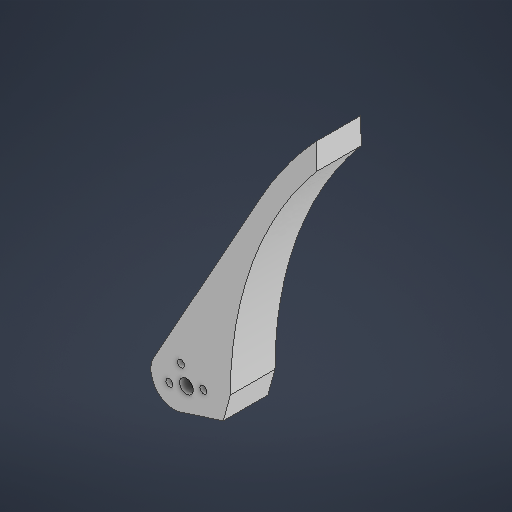
# Autodesk Inventor part: направление
Saved by Autodesk Inventor 2025 (Build 290162000, 162)
## iProperties
Created: 2025-11-04
Part Number: направление
Material: Типовые
Document SubType Name: Modeling
Designer: GameHD
Density: 1 g/cm^3
Appearance: По умолчанию
Author: GameHD
Autodesk Inventor part; units mm, degrees
ref_plane "YZ Plane" through (0, 0, 0) normal (1, 0, 0) x (0, 1, 0)
ref_plane "XZ Plane" through (0, 0, 0) normal (0, 1, 0) x (-1, 0, 0)
ref_plane "XY Plane" through (0, 0, 0) normal (0, 0, 1) x (1, 0, 0)
sketch "Эскиз1" plane through (0, 0, 0) normal (0, 0, 1) x (1, 0, 0)
  circle A0 centre (0, 0) radius 165
  circle A1 centre (0, 0) radius 172.834
  line L0 (-125, 0) -> (-126.5392, 117.7261)
  line L1 (-132.7592, 119.5177) -> (-197.8467, 76.6552)
  line L2 (-165, 0) -> (-153, 0) construction
  line L3 (-134.7038, 9.8338) -> (-172.765, -2.5204) projected
  line L4 (-165, 0) -> (-172.8154, -2.5368)
  point P0 (-172.834, 0)
  point P1 (-126.3868, 106.0725)
  point P2 (-123, 114.4334)
  point P3 (-172.8149, -2.5694)
  dimension "d0" = 330
  dimension "d1" = 345.668
  dimension "d2" = 40
  constraints: 8 end point, 4 point on circle, 2 coincident, 1 centre point, 1 collinear, 1 horizontal, 1 tangent, 3 other
  measures "d1" diameter of A1
  measures "d2" distance of L2.start L0.start
extrude "Выдавливание1" add sketch "Эскиз1" along normal blind 20 contours L3 L4 A1 L0 A0 picked at (-133.2989, 101.385)
sketch "Эскиз2" plane through (0, 0, 0) normal (0, 0, -1) x (-1, 0, 0)
  arc A0 (172.8154, -2.5368) -> (126.5392, 117.7261) centre (0, 0) ccw projected
  arc A1 (165, 0) -> (126.3868, 106.0725) centre (0, 0) ccw projected
  circle A2 centre (0, 0) radius 168.917
  line L0 (172.8154, -2.5368) -> (165, 0) projected
  circle A3 centre (184.6734, -6.3858) radius 2.1
  line L1 (178.0154, -4.2246) -> (172.8154, -2.5368)
  line L2 (160.1198, 6.946) -> (198.8648, -5.6302)
  line L3 (182.8662, -5.7992) -> (187.0032, 6.946)
  line L4 (178.0154, -4.2246) -> (198.192, -10.7737)
  line L5 (184.6734, -6.3858) -> (189.5243, -7.9603)
  line L6 (189.5243, -7.9603) -> (192.7095, 1.8528)
  point P0 (184.4408, -0.9483)
  point P1 (172.8109, 2.8266)
  point P2 (176.018, -3.5763)
  point P3 (182.676, -5.7374)
  point P4 (183.1424, -4.9484)
  point P5 (164.9119, 5.3905)
  point P6 (186.6708, -7.0341)
  point P7 (191.0988, -3.1094)
  dimension "d8" = 337.834
  dimension "d11" = 4.2
  dimension "d18" = 5.1
  constraints: 12 end point, 2 centre point, 2 perpendicular, 1 coincident, 1 collinear, 1 parallel, 1 point on line
  measures "d8" diameter of A2
  measures "d11" diameter of A3
  measures "d18" distance of L5.start L5.end
extrude "Выдавливание2" add sketch "Эскиз2" against normal up to surface (20 mm away) contours L0 A2 L2 A0 | A0 L2 L3 A3 L4 L1 | L0 A1 L2 A2 | L2 L6 L4 A3 L3 picked at (166.282, 2.7097)
sketch "Эскиз3" plane through (0, 0, 20) normal (0, 0, 1) x (1, 0, 0)
  arc A0 (-126.3868, 106.0725) -> (-165, 0) centre (0, 0) ccw projected
  line L0 (-126.3868, 106.0725) -> (-126.5392, 117.7261) projected
  arc A1 (-126.5392, 117.7261) -> (-172.8109, 2.8266) centre (0, 0) ccw projected
  line L1 (-191.0988, -3.1094) -> (-172.8109, 2.8266) projected
  line L2 (-189.5243, -7.9603) -> (-191.0988, -3.1094) projected
  line L3 (-186.6708, -7.0341) -> (-189.5243, -7.9603) projected
  arc A2 (-182.676, -5.7374) -> (-186.6708, -7.0341) centre (-184.6734, -6.3858) ccw projected
  line L4 (-165, 0) -> (-182.676, -5.7374) projected
  circle A3 centre (-184.6734, -6.3858) radius 3.1
  arc A4 (-126.5392, 117.7261) -> (-172.8109, 2.8266) centre (0, 0) ccw projected
  line L5 (-184.6734, -6.3858) -> (-194.1849, -9.4731)
  line L6 (-194.1849, -9.4731) -> (-195.7594, -4.6222)
  line L7 (-195.7594, -4.6222) -> (-191.0988, -3.1094)
  circle A5 centre (-184.6734, -6.3858) radius 11
  circle A6 centre (-184.6734, -6.3858) radius 9.5
  circle A7 centre (-184.6734, -6.3858) radius 6.5
  line L8 (-190.8559, -8.3925) -> (-193.7093, -9.3187)
  circle A8 centre (-192.2826, -8.8556) radius 1.6
  circle A9 centre (-182.2036, -13.995) radius 1.6
  circle A10 centre (-177.0642, -3.9159) radius 1.6
  circle A11 centre (-187.1433, 1.2234) radius 1.6
  line L9 (-192.2826, -8.8556) -> (-199.8918, -11.3255)
  line L10 (-199.8918, -11.3255) -> (-201.4663, -6.4746)
  line L11 (-201.4663, -6.4746) -> (-191.0988, -3.1094)
  line L12 (-201.4663, -6.4746) -> (-195.8644, -23.7333)
  line L13 (-172.8109, 2.8266) -> (-166.0857, -17.8924)
  line L14 (-184.6734, -6.3858) -> (-181.5861, -15.8973)
  line L15 (-165, 0) -> (-182.676, -5.7374) projected
  line L16 (-209.847, -25.0704) -> (-154.8396, -7.2156)
  line L17 (-201.4663, -6.4746) -> (-150.7943, 84.4559)
  line L18 (-165, 0) -> (-168.149, -11.5357)
  point P0 (-182.1957, -12.395)
  point P1 (-183.1496, -12.7046)
  point P2 (-195.5181, -4.5439)
  point P3 (-195.5997, -5.1144)
  point P4 (-193.5037, -9.8895)
  point P5 (-175.4687, -4.0356)
  point P6 (-178.5861, -4.4099)
  point P7 (-181.7249, -5.4287)
  point P8 (-187.622, -7.3428)
  point P9 (-150.9747, 84.1323)
  point P10 (-193.8045, -9.3496)
  point P11 (-196.8045, -20.837)
  point P12 (-168.149, -11.5357)
  point P13 (-171.2364, -2.0242)
  point P14 (-175.5424, -3.4219)
  point P15 (-181.1697, -15.216)
  point P16 (-182.3233, -15.5905)
  dimension "d22" = 19
  dimension "d23" = 13
  dimension "d19" = 6.2
  dimension "d20" = 10
  dimension "d21" = 22
  dimension "d24" = 3.2
  dimension "d27" = 360
  dimension "d29" = 8
  dimension "d30" = 10
  dimension "d33" = 10
  constraints: 26 end point, 6 centre point, 6 point on line, 5 perpendicular, 4 coincident, 1 midpoint, 1 parallel, 1 tangent, 15 other
  measures "d19" diameter of A3
  measures "d20" distance of L5.start L5.end
  measures "d21" diameter of A5
  measures "d24" diameter of A8
  measures "d29" distance of L9.start L9.end
  measures "d30" distance of L14.start L14.end
  measures "d33" distance from line of L16 A2.centre
extrude "Выдавливание3" add sketch "Эскиз3" against normal up to surface (20 mm away) contours A1 L1 A5 L7 L11 L17 | L11 L6 A5 L9 L10 | L1 A6 A11 L7 A5 | L13 L16 A5 L4 | L4 L18 L13 | L9 A5 L16 L12 | L7 A5 L6 | L1 A7 A11 A6 | A5 L16 L14 A9 A6 A10 L4 | L7 A6 A8 L5 L6 A5 | L9 L5 A8 A6 A9 L14 L16 A5 | A5 L6 L9 | L1 A7 A11 | A6 A11 A7 L1 L7 | L7 L2 A7 A8 A6 | L2 L5 A8 A7 | A10 A7 A9 L14 A3 L4 | A6 A9 A7 A10 | L14 A6 A9 | A9 A6 L14 | A8 A7 A9 A6 | L3 A3 L14 A9 A7 A8 L5 | A9 A7 L14 A6 | A6 L14 A7 A9 | A9 L14 A7 | L14 A9 A7
sketch "Эскиз4" plane through (0, 0, 20) normal (0, 0, 1) x (1, 0, 0)
  arc A0 (-187.622, -7.3428) -> (-181.7249, -5.4287) centre (-184.6734, -6.3858) ccw projected
  arc A1 (-178.5861, -4.4099) -> (-175.5424, -3.4219) centre (-177.0642, -3.9159) ccw projected
  circle A2 centre (-184.6734, -6.3858) radius 3.1
  circle A3 centre (-177.0642, -3.9159) radius 1.6
  point P0 (0, 0)
  point P1 (-175.5424, -3.4219)
  point P2 (-178.5861, -4.4099)
  point P3 (-181.7249, -5.4287)
  point P4 (-187.622, -7.3428)
  constraints: 2 centre point, 2 coincident, 2 concentric
extrude "Выдавливание4" cut sketch "Эскиз4" against normal through all
fillet "Сопряжение2" radius 10 2 edges at (-201.4663, -6.4746, 10) (-196.8045, -20.837, 10)
